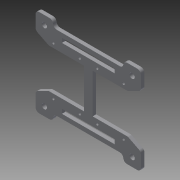
# Autodesk Inventor part: odometer_base
Saved by Autodesk Inventor 2014 SP1 (Build 180222100, 222)
## iProperties
Created: 2015-07-19
Part Number: odometer_base
Material: Générique
Document SubType Name: Modeling
Designer: astralien3000
Density: 1 g/cm^3
Appearance: Par défaut
Author: astralien3000
Autodesk Inventor part; units mm, degrees
ref_plane "YZ Plane" through (0, 0, 0) normal (1, 0, 0) x (0, 1, 0)
ref_plane "XZ Plane" through (0, 0, 0) normal (0, 1, 0) x (-1, 0, 0)
ref_plane "XY Plane" through (0, 0, 0) normal (0, 0, 1) x (1, 0, 0)
sketch "Esquisse1" plane through (0, 0, 0) normal (0, 1, 0) x (-1, 0, 0)
  line L0 (0, 0) -> (50, 0) construction
  line L1 (50, 0) -> (50, 40) construction
  line L2 (50, 40) -> (0, 40) construction
  line L3 (0, 40) -> (0, 0) construction
  circle A0 centre (50, 40) radius 3
  line L4 (0, 50) -> (5, 50)
  line L5 (5, 50) -> (5, 0)
  line L6 (5, 0) -> (0, 0)
  line L7 (0, 0) -> (0, 50)
  line L8 (5, 22.5) -> (45, 22.5)
  line L9 (45, 22.5) -> (45, 50)
  line L10 (45, 50) -> (5, 50)
  line L11 (5, 50) -> (5, 22.5)
  line L12 (45, 22.5) -> (5, 22.5)
  line L13 (5, 22.5) -> (5, 32.5)
  line L14 (5, 32.5) -> (45, 32.5) construction
  line L15 (45, 32.5) -> (45, 22.5)
  line L16 (35, 32.5) -> (45, 32.5) construction
  line L17 (45, 32.5) -> (45, 22.5) construction
  line L18 (45, 22.5) -> (35, 22.5) construction
  line L19 (35, 22.5) -> (35, 32.5) construction
  line L20 (15, 22.5) -> (5, 22.5) construction
  line L21 (5, 22.5) -> (5, 32.5) construction
  line L22 (5, 32.5) -> (15, 32.5) construction
  line L23 (15, 32.5) -> (15, 22.5) construction
  line L24 (5, 22.5) -> (15, 32.5) construction
  line L25 (5, 32.5) -> (15, 22.5) construction
  line L26 (45, 32.5) -> (35, 22.5) construction
  line L27 (35, 32.5) -> (45, 22.5) construction
  circle A1 centre (10, 27.5) radius 1.5
  circle A2 centre (40, 27.5) radius 1.5
  line L28 (45, 50) -> (60, 50)
  line L29 (60, 50) -> (60, 30)
  line L30 (60, 30) -> (45, 30)
  line L31 (45, 30) -> (45, 50)
  line L32 (45, 22.5) -> (60, 30)
  dimension "d0" = 40
  dimension "d1" = 50
  dimension "d2" = 6
  dimension "d3" = 45
  dimension "d4" = 40
  dimension "d5" = 22.5
  dimension "d7" = 10
  dimension "d8" = 5
  dimension "d11" = 10
  dimension "d12" = 10
  dimension "d13" = 10
  dimension "d14" = 3
  dimension "d15" = 3
  dimension "d33" = 60
  dimension "d34" = 10
  constraints: 66 end point, 14 parallel, 7 horizontal, 7 perpendicular, 6 point on line, 3 centre point, 2 midpoint, 1 coincident, 1 collinear
  measures "d0" distance of L2.end L0.start
  measures "d1" distance of L0.start L0.end
  measures "d2" diameter of A0
  measures "d3" distance between parallel lines of L7 L9
  measures "d4" distance between parallel lines of L9 L5
  measures "d5" distance between parallel lines of L0 L8
  measures "d7" distance from line of L10 L1.end
  measures "d8" distance from line of L9 L1.end
  measures "d11" distance between parallel lines of L12 L14
  measures "d12" distance between parallel lines of L21 L23
  measures "d13" distance between parallel lines of L9 L19
  measures "d14" diameter of A1
  measures "d15" diameter of A2
  measures "d33" distance between parallel lines of L7 L29
  measures "d34" distance from line of L1.end L30
extrude "Extrusion1" add sketch "Esquisse1" along normal blind 4
mirror "Symétrie1" about plane through (0, 0, 0) normal (0, 0, 1) of "Extrusion1"
mirror "Symétrie2" about plane through (0, 0, 0) normal (1, 0, 0) of "Extrusion1"
mirror "Symétrie3" about plane through (0, 0, 0) normal (0, 0, 1) of "Extrusion1", "Symétrie2"
sketch "Esquisse2" plane through (0, 4, 0) normal (0, 1, 0) x (1, 0, 0)
  circle A0 centre (50, 40) radius 3 projected
  circle A1 centre (-50, 40) radius 3 projected
  line L0 (60, 50) -> (-60, 50) projected
  line L1 (0, 0) -> (0, 50) construction
  line L2 (40, 50) -> (-40, 50)
  line L3 (-30, 37.5) -> (30, 37.5)
  line L4 (30, 37.5) -> (30, 32.5)
  line L5 (30, 32.5) -> (-30, 32.5)
  line L6 (-30, 32.5) -> (-30, 37.5)
  line L7 (-40, 50) -> (40, 50)
  line L8 (40, 50) -> (40, 42.5)
  line L9 (40, 42.5) -> (-40, 42.5)
  line L10 (-40, 42.5) -> (-40, 50)
  circle A2 centre (10, 27.5) radius 1.5 projected
  point P0 (45, 60)
  point P1 (-45, 60)
  point P2 (0, 50)
  dimension "d24" = 30
  dimension "d25" = 30
  dimension "d26" = 5
  dimension "d28" = 10
  dimension "d29" = 10
  dimension "d30" = 5
  dimension "d31" = 5
  constraints: 20 end point, 4 parallel, 3 horizontal, 2 perpendicular, 1 coincident, 1 midpoint, 3 other
  measures "d24" distance between parallel lines of L1 L4
  measures "d25" distance between parallel lines of L6 L1
  measures "d26" distance between parallel lines of L3 L5
  measures "d28" horizontal distance of L2.start A0.centre
  measures "d29" horizontal distance of L2.end A1.centre
  measures "d30" distance between parallel lines of L9 L3
  measures "d31" distance from line of L5 A2.centre
extrude "Extrusion2" cut sketch "Esquisse2" against normal through all contours L8 L9 L10 L0 | L3 L4 L5 L6
mirror "Symétrie4" about plane through (0, 0, 0) normal (0, 0, 1) of "Extrusion2"
fillet "Congé1" radius 4 20 edges at (-40, 2, -50) (40, 2, 50) (40, 2, 42.5) (-40, 2, 50) (-40, 2, 42.5) (40, 2, -50) (-40, 2, -42.5) (40, 2, -42.5) (60, 2, -50) (60, 2, -30) (45, 2, -22.5) (-60, 2, -50) (-60, 2, -30) (-45, 2, -22.5) (-45, 2, 22.5) (-60, 2, 30) (-60, 2, 50) (60, 2, 50) (60, 2, 30) (45, 2, 22.5)
equation "\"d12\" = d11"
equation "\"d13\" = d11"
equation "\"d34\" = d7"
equation "\"d25\" = d24"
